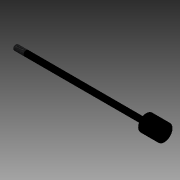
# Autodesk Inventor part: C-044-DP0000_rod
Saved by Autodesk Inventor 2014 SP2 (Build 180246200, 246)
## iProperties
Created: 2020-02-04
Part Number: C-044-DP0000_rod
Material: Generic
Catalog Web Link: www.cadenas.de
Description: Standard Air Cylinder_rod-Original Line - Standard Air Cylinders
Vendor: BIMBA
Document SubType Name: Modeling
Designer: psadmin
Manufacturer: BIMBA
Mass: 11.131 g
Surface Area: 49.6781 cm^2
Volume: 11.131 cm^3
Density: 1 g/cm^3
Appearance: PSOLRGB-0-0-0
Category: PARTsolutions
Company: BIMBA
Title: C-044-DP0000_rod
Author: Cadenas PARTsolutions
Comments: Original Line - Standard Air Cylinders
PSOL_IDENT_0: {$CADENAS_DATA\23d-libs\bimba\bimba_brand\bimba_imperial\bimba_full_line\original_line_cylinders\sta
PSOL_IDENT_1: ndard_air_cylinders\rod.prj},333 {VTYP=3D},{NB=C-044-DP0000_rod},{LINA=C-044-DP0000_rod},{NN=Standar
PSOL_IDENT_2: d Air Cylinder_rod},{DATE=22.01.2020 09:07:35},{GEOMDATE=27.08.2019 11:00:52},{VERSION=},{LINEID=50}
PSOL_IDENT_3: ,{WBVAR=STROKE,ACTING,MNT,DER,NR,BM,CO,M,EE,EEL,K,Q,Y,F,G,T,B,H,SER,SR,NT,W,E,HL,ST,STP,PRC,PB,COLOR
PSOL_IDENT_4: 1,FCD,RCD,BCD,ZHJ},{WBNUMERIC=STROKE,EEL,COLOR1,FCD,RCD,BCD,ZHJ}  {NB=C-044-DP0000_rod},{LINA=C-044-
PSOL_IDENT_5: DP0000_rod},{KT=DUMMY},{PN=C-044-DP000},{DASH=-},{BORE=0.75000000},{BOREPN=04},{STROKE=4.000},{STROK
PSOL_IDENT_6: EALG=[0.001:50/0.001]},{STROKE1=4.000},{ACTING=D},{ACTINGALG= '' , 'Single Acting' , 'R' , 'Reverse
PSOL_IDENT_7: Single Acting' , 'D' , 'Double Acting' },{ACTINGPN=D},{MNT=P},{MNTALG= '' , 'Front Nose Mounting' , '
PSOL_IDENT_8: P' , 'Rear Pivot Mounting' , 'XP' , 'Double End or Pivot Mounting' , 'X' , 'Double End Mounting' , '
PSOL_IDENT_9: BF' , 'Front Block Mounting' , 'BR' , 'Rear Block Mounting for Vertical Positioning' , 'BFT' , 'Fron
PSOL_IDENT_10: t Block Trunnion Mounting' , 'BRT' , 'Rear Block Trunnion Mounting' },{TYPE=C-},{MNTPN=P},{DER=},{DE
PSOL_IDENT_11: RALG= '' , 'N/A' },{NR=},{NRALG= '' , 'N/A' },{NRPN=},{BM=},{BMALG= '' , 'N/A' },{BMPN=},{CO=},{COAL
PSOL_IDENT_12: G= '' , 'N/A' },{M=},{MALG= '', 'Without Magnet', 'M', 'With Magnet' },{EE=},{EEL=0},{EEMAX=8},{EEAL
PSOL_IDENT_13: G= '', 'Without Extra Extension', 'EE', 'With Extra Extension' },{EELALG=0},{EEPN=},{EEPN1=0.000},{K=
PSOL_IDENT_14: },{KALG= '', 'Standard' , 'K' , 'Ports Rotated 90deg' },{KPN=},{Q=},{QALG= '' , 'Without Side Ported
PSOL_IDENT_15: Rear Head' , 'Q' , 'With Side Ported Rear Head' },{QPN=},{Y=},{YALG= '' , 'Without Pivot Bushing' ,
PSOL_IDENT_16: 'Y' , 'With Pivot Bushing' },{YPN=},{F=},{FALG= '', 'Standard', 'F', 'Molycoated Body' },{FPN=},{G=
PSOL_IDENT_17: },{GPN=},{T=},{TALG= '' , 'Standard' , 'N' , 'Low Temperature' , 'V' , 'High Temperature' },{NPN=},{
PSOL_IDENT_18: VPN=},{B=},{BALG= '', 'Without Bumper' , 'B' , 'With Bumper' },{BPN=},{H=},{HALG= '', 'N/A' },{HPN=}
PSOL_IDENT_19: ,{SER=},{SERALG= '' , 'Without Spring Extend/Return' , 'JS' , 'With Spring Return' , 'JR' , 'With Sp
PSOL_IDENT_20: ring Extend' },{SR=C},{SRALG= 'C' , 'Carbon Steel Rod' , 'SR' , '303 Stainless Steel Rod' , '' , '30
PSOL_IDENT_21: 3 Stainless Steel Rod1' },{SRPN=C},{SRCON=1},{NT=},{NTPN=},{W=},{WALG= '' , 'Without Wiper' , 'W' , '
PSOL_IDENT_22: With Wiper' },{WPN=},{E=},{EALG= '' , 'Without Special Lube and Seals' , 'E' , 'With Special Lube an
PSOL_IDENT_23: d Seals' },{EPN=},{HL=},{HLALG= '' , 'Wihout Low Pressure Hydraulic' , 'HL' , 'With Low Pressure Hyd
PSOL_IDENT_24: raulic' },{ST=},{STALG= '' , 'Without Switch Track' , 'T' , 'With Switch Track' },{STP=},{STPALG= ''
PSOL_IDENT_25: , 'N/A' },{STPN=},{PRC=},{PRCALG= '' , 'Without Piston Rod Clevis' , 'D-166-1' , 'With Piston Rod C
PSOL_IDENT_26: levis' },{PRCPN=},{PB=},{PBALG= '' , 'Without Pivot Bracket' , 'D-167' , 'With Pivot Bracket' },{PBP
PSOL_IDENT_27: N=},{TLEN=5.2555},{TEXT=0.366667},{SPACE=0.209524},{FRAC=22.7500},{RGCON=},{RGDACCON=R},{RHCON=P},{R
PSOL_IDENT_28: HCONON=1},{RHACCON=},{FNUTCON=0},{RNUTCON=0},{FNUTPN=},{RNUTPN=},{FNUTTRANS=0.0000},{RNUTTRANS=0.000
PSOL_IDENT_29: 0},{VHOLECON=0},{A1=1.5940},{A1N=0.8750},{A1P=1.5940},{A1B=1.5940},{A4=0.2525},{A4N=0.3130},{A4P=0.2
PSOL_IDENT_30: 525},{A5=0.0300},{A1H=1.594},{A1NH=0.5310},{A1PH=1.5940},{A1BH=1.0940},{A1SH=1.2190},{A2H=0.2190},{A
PSOL_IDENT_31: 2NH=0.2190},{LENGTH=3.7500},{LENGTH1=3.7500},{LENGTH2=3.8100},{MUL=4.0000},{MUL11=4.0000},{MUL22=10.
PSOL_IDENT_32: 7600},{MUL33=6.7600},{MUL2=4.0000},{MUL211=4.0000},{MUL222=2.6900},{MUL233=1.6900},{SSS=8.0000},{RGL
PSOL_IDENT_33: EN=1.3715},{RHLEN=1.1230},{SSS1=5.0000},{A13=1.3120},{THDLEN1=0.5000},{THD1=0.2500},{TAB=UNF},{THDLE
PSOL_IDENT_34: N=0.5000},{THD=0.2500},{OD=0.7615},{RODL=6.9380},{PL=0.8440},{RODDIA=0.2500},{HEX=0.2500},{RODTRANS=
PSOL_IDENT_35: 0.0000},{G1=0.1250},{ON=0},{G5=0.6250},{DERLEN=6.0940},{THOLE=0.0000},{WF=0.2200},{BADD=0.0000},{MAD
PSOL_IDENT_36: D=0.0000},{NVADD=0.000},{JRADD=0.00000},{COLOR=0.00,0.00,0.00,0.00},{GROOVE=1},{HOL=0},{D7=0.2520},{
PSOL_IDENT_37: H1=1.1175},{D1=0.8625},{D1RH=0.8625},{D1P=0.8325},{D1B=0.8625},{D1N=0.8050},{D1NRH=0.8050},{D1BRH=0.
PSOL_IDENT_38: 8325},{D1PRH=0.8625},{BOZO=0},{HADD=0.000},{COLOR1=0},{DEFL=0.0000},{HEXL=0.0000},{SSADD=0.0000},{WF
PSOL_IDENT_39: L=0.0000},{MOVE=0.0000},{PRCL2=0.50000},{PRCB=0.16000},{PRCTRANS=0.16000},{FCD=0},{RCD=0},{BCD=0},{Z
PSOL_IDENT_40: HJ=0.000}
NN: Standard Air Cylinder_rod
NT: Standard
NB: C-044-DP0000_rod
NBSYN: $PN.$COLOR1._rod
LINA: C-044-DP0000_rod
PN: C-044-DP000
BORE: 0.75
BOREPN: 04
STROKE: 4
ACTING: Double Acting
MNT: Rear Pivot Mounting
DER: N/A
NR: N/A
BM: N/A
CO: N/A
M: Without Magnet
EE: Without Extra Extension
EEL: 0
K: Standard
Q: Without Side Ported Rear Head
Y: Without Pivot Bushing
F: Standard
G: Without Magnalube Lubrication
T: Standard
B: Without Bumper
H: N/A
SER: Without Spring Extend/Return
SR: Carbon Steel Rod
W: Without Wiper
E: Without Special Lube and Seals
HL: Wihout Low Pressure Hydraulic
ST: Without Switch Track
STP: N/A
PRC: Without Piston Rod Clevis
PB: Without Pivot Bracket
A1N: 0.875
A1P: 1.594
A1B: 1.594
A4N: 0.313
A4P: 0.2525
A5: 0.03
A1NH: 0.531
A1PH: 1.594
A1BH: 1.094
A1SH: 1.219
A2NH: 0.219
A13: 1.312
THDLEN1: 0.5
THD1: 0.25
TAB: UNF
OD: 0.7615
RODDIA: 0.25
HEX: 0.25
G1: 0.125
G5: 0.625
THOLE: 0
WF: 0.22
GROOVE: 1
D7: 0.252
D1P: 0.8325
D1B: 0.8625
D1N: 0.805
D1NRH: 0.805
D1BRH: 0.8325
D1PRH: 0.8625
COLOR1: 0
FCD: 0
RCD: 0
BCD: 0
ZHJ: 0
SUPPLIER: BIMBA
ARTICLENO: C-044-DP0000_rod
BOMINFO: C-044-DP0000_rod
CREATOR: CADENAS GmbH
Autodesk Inventor part; units mm, degrees
sketch "Sketch_1" plane through (0, 0, 0) normal (0, 0, 1) x (1, 0, 0)
  line L0 (163.5252, 0) -> (0, 0)
  line L1 (0, 0) -> (0, 3.175)
  line L2 (0, 3.175) -> (142.0876, 3.175)
  line L3 (142.0876, 3.175) -> (142.0876, 9.6203)
  line L4 (142.0876, 9.6203) -> (163.5252, 9.6203)
  line L5 (163.5252, 9.6203) -> (163.5252, 0)
  line L6 (163.5252, 0) -> (0, 0)
  constraints: 14 end point
revolve "Revolution1" add sketch "Sketch_1" angle 360 about axis through (163.5252, 0, 0) along (1, 0, 0)
sketch "Sketch_3" plane through (0, 0, 0) normal (0, 0, 1) x (1, 0, 0)
  line L0 (0, 0) -> (-12.7, 0)
  line L1 (-12.7, 0) -> (-12.7, 2.634)
  line L2 (-12.7, 2.634) -> (-12.159, 3.175)
  line L3 (-12.159, 3.175) -> (0, 3.175)
  line L4 (0, 3.175) -> (0, 0)
  line L5 (0, 0) -> (-12.7, 0)
  constraints: 12 end point
revolve "Revolution2" add sketch "Sketch_3" angle 360 about axis through (0, 0, 0) along (1, 0, 0)
thread "Thread1" size "1/4-28 UNF" class "2A" standard "ANSI Unified Screw Threads" length 12.159
sketch "Sketch_30" plane through (0, 0, 0) normal (0, 0, 1) x (1, 0, 0)
  line L0 (0, 0) -> (-0.254, 0)
  line L1 (-0.254, 2.921) -> (0, 2.921)
  line L2 (0, 2.921) -> (0, 3.429)
  line L3 (0, 3.429) -> (-0.254, 3.429)
  line L4 (-0.254, 3.429) -> (-0.254, 2.921)
  constraints: 10 end point
revolve "Revolution3" cut sketch "Sketch_30" angle 360 about axis through (0, 0, 0) along (1, 0, 0)
ref_plane "dia1_XY" through (0, 3.175, 0) normal (1, 0, 0) x (0, 0, -1)
ref_plane "dia1_YZ" through (0, 3.175, 0) normal (0, 0, -1) x (0, 1, 0)
ref_plane "dia1_ZX" through (0, 3.175, 0) normal (0, 1, 0) x (1, 0, 0)
ref_plane "dia12_XY" through (0, 0, 10.9537) normal (1, 0, 0) x (0, 0, -1)
ref_plane "dia12_YZ" through (0, 0, 10.9537) normal (0, 0, -1) x (0, 1, 0)
ref_plane "dia12_ZX" through (0, 0, 10.9537) normal (0, 1, 0) x (1, 0, 0)
ref_plane "dia2_XY" through (0, -3.175, 0) normal (1, 0, 0) x (0, 0, -1)
ref_plane "dia2_YZ" through (0, -3.175, 0) normal (0, 0, -1) x (0, 1, 0)
ref_plane "dia2_ZX" through (0, -3.175, 0) normal (0, 1, 0) x (1, 0, 0)
ref_plane "dia22_XY" through (0, 0, -10.9537) normal (1, 0, 0) x (0, 0, -1)
ref_plane "dia22_YZ" through (0, 0, -10.9537) normal (0, 0, -1) x (0, 1, 0)
ref_plane "dia22_ZX" through (0, 0, -10.9537) normal (0, 1, 0) x (1, 0, 0)
ref_plane "rl1_XY" through (-12.7, 0, 0) normal (1, 0, 0) x (0, 0, -1)
ref_plane "rl1_YZ" through (-12.7, 0, 0) normal (0, 0, -1) x (0, 1, 0)
ref_plane "rl1_ZX" through (-12.7, 0, 0) normal (0, 1, 0) x (1, 0, 0)
ref_plane "rl2_XY" through (0, 0, 0) normal (1, 0, 0) x (0, 0, -1)
ref_plane "rl2_YZ" through (0, 0, 0) normal (0, 0, -1) x (0, 1, 0)
ref_plane "rl2_ZX" through (0, 0, 0) normal (0, 1, 0) x (1, 0, 0)
ref_plane "rod_cp_XY" through (0, 0, 0) normal (1, 0, 0) x (0, 0, -1)
ref_plane "rod_cp_YZ" through (0, 0, 0) normal (0, 0, -1) x (0, 1, 0)
ref_plane "rod_cp_ZX" through (0, 0, 0) normal (0, 1, 0) x (1, 0, 0)
ref_plane "thd1_XY" through (-12.7, 3.175, 0) normal (1, 0, 0) x (0, 0, -1)
ref_plane "thd1_YZ" through (-12.7, 3.175, 0) normal (0, 0, -1) x (0, 1, 0)
ref_plane "thd1_ZX" through (-12.7, 3.175, 0) normal (0, 1, 0) x (1, 0, 0)
ref_plane "thd2_XY" through (-12.7, -3.175, 0) normal (1, 0, 0) x (0, 0, -1)
ref_plane "thd2_YZ" through (-12.7, -3.175, 0) normal (0, 0, -1) x (0, 1, 0)
ref_plane "thd2_ZX" through (-12.7, -3.175, 0) normal (0, 1, 0) x (1, 0, 0)
ref_plane "to_rod_clevis_XY" through (-16.764, 0, 0) normal (1, 0, 0) x (0, 0, -1)
ref_plane "to_rod_clevis_YZ" through (-16.764, 0, 0) normal (0, 0, -1) x (0, 1, 0)
ref_plane "to_rod_clevis_ZX" through (-16.764, 0, 0) normal (0, 1, 0) x (1, 0, 0)
body "Solid1"
